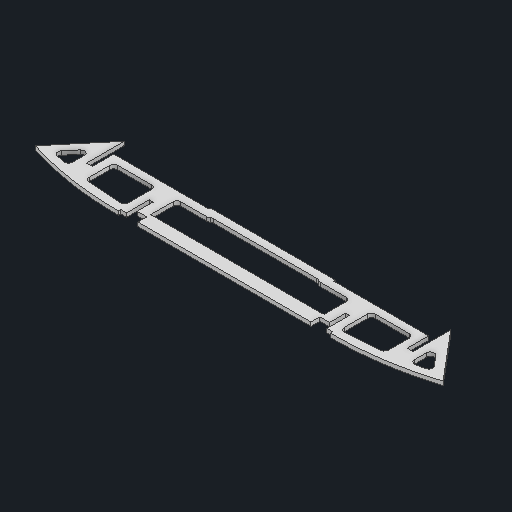
# Autodesk Inventor part: tail_2
Saved by Autodesk Inventor 2023 (Build 270158030, 158C)
## iProperties
Created: 2022-03-21
Part Number: tail_2
Material: Generic
Document SubType Name: Modeling
Designer: kardo
Density: 1 g/cm^3
Appearance: Default
Author: kardo
Autodesk Inventor part; units mm, degrees
ref_plane "YZ Plane" through (0, 0, 0) normal (1, 0, 0) x (0, 1, 0)
ref_plane "XZ Plane" through (0, 0, 0) normal (0, 1, 0) x (-1, 0, 0)
ref_plane "XY Plane" through (0, 0, 0) normal (0, 0, 1) x (1, 0, 0)
derived "parameters_frame.ipt"
derived "stencil_frame.ipt"
sketch "sk_joint_locations" plane through (81.12, 0, 0) normal (1, 0, 0) x (0, 1, 0)
  line L0 (0, 0) -> (111.39, 7.7891) construction
  line L1 (30.81, 28.832) -> (94.8, 28.832) construction
  arc A0 (30.81, 28.832) -> (9.48, 28.5282) centre (30.81, -720.1791) ccw construction
  line L2 (-254.1001, 21.0191) -> (9.48, 28.5282) construction
  line L3 (-363, 18.496) -> (-275.8801, 20.463) construction
  arc A1 (-275.8801, 20.463) -> (-254.1001, 21.0191) centre (-359.1231, 3707.4463) ccw construction
  line L4 (-210.8824, 4616.4994) -> (225.0382, -1617.4555) construction
  line L5 (-242.0001, 4592.9714) -> (-242.0001, -1605.7041) construction
  line L6 (-120.9999, 4592.9714) -> (-120.9999, -1605.7041) construction
  line L7 (-363, 4592.9714) -> (-363, -1605.7041) construction
  line L8 (0, 4592.9714) -> (0, -1605.7041) construction
  line L9 (551.8244, 47.4419) -> (-603.6686, 7.0912) construction
  line L10 (-657.8036, -26.1228) -> (709.4042, 69.4817) construction
  line L11 (178.2183, 30.3929) -> (177.9391, 38.388) construction
  line L12 (185.9231, 36.8959) -> (186.4825, 28.8959) construction
  line L13 (0, 6.528) -> (111.1168, 11.6964) construction
  line L14 (-242.0001, 45.8501) -> (-242.0001, 21.3638) construction
  line L15 (-363, 37.4293) -> (-363, 18.496) construction
  line L16 (-120.9999, 51.0063) -> (-120.9999, 24.811) construction
  line L17 (0, 52.89) -> (0, 28.2581) construction
  line L18 (108.3896, 50.6971) -> (108.935, 42.897) construction
  line L19 (109.4805, 35.0968) -> (108.935, 42.897) construction
  line L20 (109.4805, 35.0968) -> (110.0259, 27.2967) construction
  line L21 (110.0259, 27.2967) -> (110.5713, 19.4965) construction
  line L22 (110.5713, 19.4965) -> (111.1168, 11.6964) construction
  line L23 (0, 6.528) -> (0, 0) construction
  spline S0 degree 4 poles (-363, 37.4293) (-272.3626, 45.1427) (-181.5879, 49.7528) (-90.8131, 52.89) (0, 52.89) knots 0 0 0 0 0 1 1 1 1 1
  spline S1 degree 3 poles (0, 52.89) (86.3106, 52.89) (181.3207, 49.5034) (237, 36.448) knots 0 0 0 0 1 1 1 1
  spline S2 degree 2 poles (111.39, 7.7891) (176.0348, 12.3096) (237, 36.448) knots 0 0 0 1 1 1
  line L24 (94.8, 37.536) -> (94.8, 28.832) construction
  line L25 (94.8, 35.548) -> (94.8, 30.82) construction
  point P0 (-210.8824, 4616.4994)
  point P1 (225.0382, -1617.4555)
  point P2 (178.0787, 34.3904)
  point P3 (186.2028, 32.8959)
  point P4 (134.9575, 11.3411)
  point P5 (-363, 27.9627)
  point P6 (-242.0001, 33.6069)
  point P7 (-120.9999, 37.9086)
  point P8 (0, 40.5741)
  point P9 (94.8, 33.184)
sketch "sk_cowl_joint_locations" plane through (54.6, 0, 0) normal (1, 0, 0) x (0, 1, 0)
  line L0 (-363, 18.496) -> (-275.8801, 20.463) construction
  arc A0 (-275.8801, 20.463) -> (-254.1001, 21.0191) centre (-359.1231, 3707.4463) ccw construction
  line L1 (-254.1001, 21.0191) -> (9.48, 28.5282) construction
  arc A1 (30.81, 28.832) -> (9.48, 28.5282) centre (30.81, -720.1791) ccw construction
  line L2 (30.81, 28.832) -> (94.8, 28.832) construction
  line L3 (94.8, 30.032) -> (30.81, 30.032) construction
  arc A2 (30.81, 30.032) -> (9.4458, 29.7277) centre (30.81, -720.1791) ccw construction
  line L4 (9.4458, 29.7277) -> (-254.1343, 22.2186) construction
  arc A3 (-275.9072, 21.6626) -> (-254.1343, 22.2186) centre (-359.1231, 3707.4463) ccw construction
  line L5 (-275.9072, 21.6626) -> (-363, 19.6963) construction
  line L6 (-242.0001, 4592.9714) -> (-242.0001, -1605.7041) construction
  line L7 (-120.9999, 4592.9714) -> (-120.9999, -1605.7041) construction
  line L8 (-363, 4592.9714) -> (-363, -1605.7041) construction
  line L9 (0, 4592.9714) -> (0, -1605.7041) construction
  line L10 (-242.0001, 45.0688) -> (-242.0001, 22.5643) construction
  line L11 (-120.9999, 49.9661) -> (-120.9999, 26.0115) construction
  line L12 (-363, 19.6963) -> (-363, 19.6963)
  line L13 (-363, 19.6963) -> (-363, 36.9211) construction
  line L14 (-1229.7832, 4422.8213) -> (280.3081, -1633.8241) construction
  line L15 (-362.7741, 36.9211) -> (-363, 39.712) construction
  line L16 (0, 51.6) -> (0, 29.4586) construction
  spline S0 degree 2 poles (-363, 39.712) (-181.6483, 54.394) (0, 54.4) knots 0 0 0 1 1 1
  spline S1 degree 3 poles (0, 54.4) (31.284, 54.4) (68.256, 47.9917) (94.8, 37.536) knots 1 1 1 1 2 2 2 2
  spline S2 degree 3 poles (93.7738, 34.9308) (89.4268, 36.6431) (81.2968, 39.4556) (71.234, 42.2519) (63.4432, 44.1558) (58.1419, 45.3261) (51.4169, 46.6598) (45.9725, 47.6212) (39.1225, 48.6857) (33.6211, 49.4253) (26.7536, 50.2046) (21.2812, 50.7098) (14.5037, 51.1886) (7.8073, 51.5121) (2.5751, 51.6) (0, 51.6) knots 1 1 1 1 1.166667 1.291667 1.333333 1.416667 1.458333 1.541667 1.583333 1.666667 1.708333 1.791667 1.833333 1.916667 2 2 2 2
  spline S3 degree 3 poles (0, 51.6) (-20.1706, 51.5993) (-55.4643, 51.3605) (-95.7903, 50.6123) (-126.0307, 49.8474) (-146.1889, 49.2356) (-171.3841, 48.3435) (-191.5382, 47.528) (-216.7283, 46.3813) (-236.8783, 45.3621) (-262.0632, 43.9608) (-282.2091, 42.7379) (-307.3889, 41.082) (-332.5661, 39.2987) (-352.7052, 37.7363) (-362.7741, 36.9211) knots 0 0 0 0 0.166667 0.291667 0.333333 0.416667 0.458333 0.541667 0.583333 0.666666 0.708333 0.791666 0.833333 0.916666 1 1 1 1
  line L17 (-142.5135, 45.4866) -> (-137.5404, 25.5402) construction
  line L18 (-134.9025, 31.4945) -> (-138.7836, 30.5268) construction
  line L19 (-137.3891, 41.4677) -> (-141.2702, 40.5) construction
  line L20 (-142.5135, 45.4866) -> (-138.6324, 46.4543) construction
  line L21 (-137.5404, 25.5402) -> (-133.6592, 26.5079) construction
  line L22 (-138.6324, 46.4543) -> (-138.8117, 52.2515) construction
  point P0 (0, 0)
  point P1 (-363, 28.3087)
  point P2 (-242.0001, 33.8165)
  point P3 (-120.9999, 37.9888)
  point P4 (0, 40.5293)
  point P5 (-1229.7832, 4422.8213)
  point P6 (280.3081, -1633.8241)
  point P7 (-85.2629, 50.788)
  point P8 (0, 40.5293)
sketch "sk_tail_2_base" plane through (0, -242.0001, 0) normal (0, 1, 0) x (-1, 0, 0)
  spline S0 degree 2 poles (-54.6, 47.8729) (-109.262, 47.8729) (-156, 14.7183) knots 0 0 0 1 1 1 construction
  line L0 (0, 47.8729) -> (-54.6, 47.8729) construction
  line L1 (760.5328, -994.3388) -> (-2384.0852, 2753.2711) construction
  line L2 (0, -1605.7041) -> (0, 4592.9714) construction
  line L3 (0, 21.7168) -> (-32.32, 21.7168)
  line L4 (-32.32, 21.7168) -> (-32.32, 22.5638)
  line L5 (-32.32, 22.5638) -> (-81.12, 22.5638)
  line L6 (-81.12, 22.5638) -> (-81.12, 33.6069)
  line L7 (-81.12, 33.6069) -> (-84.12, 33.6069)
  line L8 (-84.12, 33.6069) -> (-84.12, 14.1461)
  line L9 (-84.12, 14.1461) -> (-105.0165, 39.0496)
  line L10 (0, 46.6729) -> (-54.6, 46.6729)
  line L11 (0, 46.6729) -> (0, 21.7168)
  spline S1 degree 5 poles (-54.6, 46.6729) (-65.235, 46.6727) (-75.8695, 45.884) (-86.4273, 44.246) (-107.4395, 39.1871) (-127.368, 30.8129) (-137.094, 25.7751) (-146.4079, 20.0514) (-155.3057, 13.7395) knots 0 0 0 0 0 0 0.493638 0.493638 0.493638 1 1 1 1 1 1
  point P0 (0, 0)
  point P1 (-34.32, 21.3638)
  point P2 (-34.32, 20.5168)
  dimension "d3" = 1.2
  dimension "d4" = 1.2
  dimension "d5" = 1.2
  dimension "d6" = 2
  dimension "d7" = 3
  dimension "d8" = 1.2
  constraints: 18 end point, 5 parallel, 4 perpendicular, 2 point on line, 1 coincident, 4 other
  measures "d4" distance from line of L3 point (-34.32, 20.517)
  measures "d5" distance from line of L5 point (-34.32, 21.364)
  measures "d6" distance from line of point (-34.32, 21.364) L4
  measures "d7" distance of L6.end L7.end
  measures "d8" distance between parallel lines of L1 L9
extrude "thicken" add sketch "sk_tail_2_base" along normal blind 2
sketch "sk_cut_joint" plane through (0, -242.0001, 0) normal (0, 1, 0) x (-1, 0, 0)
  line L0 (0, 47.8729) -> (-54.6, 47.8729) projected
  line L1 (-54.6, -1605.7041) -> (-54.6, 4592.9714) construction
  line L2 (-49.6, 47.8729) -> (-49.6, 33.8165)
  line L3 (-49.6, 33.8165) -> (-51.6, 33.8165)
  line L4 (-51.6, 33.8165) -> (-51.6, 47.8729)
  point P0 (0, 0)
  point P1 (-54.6, 33.8165)
  dimension "d11" = 5
  dimension "d12" = 2
  constraints: 6 end point, 3 parallel, 3 point on line
  measures "d11" distance between parallel lines of L1 L2
  measures "d12" distance between parallel lines of L2 L4
extrude "cut_joint" cut sketch "sk_cut_joint" along normal through all both and the other way through all
sketch "sk_cut_liner" plane through (0, -242.0001, 0) normal (0, 1, 0) x (-1, 0, 0)
  line L0 (0, 47.8729) -> (-54.6, 47.8729) projected
  line L1 (-54.6, -1605.7041) -> (-54.6, 4592.9714) projected
  line L2 (-44.6, 47.8729) -> (-44.6, 42.0729)
  line L3 (-44.6, 42.0729) -> (-49.6, 42.0729)
  line L4 (-49.6, 42.0729) -> (-49.6, 45.4729)
  line L5 (-49.6, 45.4729) -> (-54.6, 45.4729)
  point P0 (0, 0)
  dimension "d14" = 2.4
  dimension "d15" = 5
  dimension "d17" = 5
  dimension "d40" = 5.8
  constraints: 8 end point, 4 parallel, 2 point on line
  measures "d14" distance between parallel lines of L0 L5
  measures "d15" distance between parallel lines of L1 L4
  measures "d17" distance between parallel lines of L2 L4
  measures "d40" distance of L2.start L2.end
extrude "cut_liner" cut sketch "sk_cut_liner" along normal through all both and the other way through all
sketch "sk_cut_weight" plane through (0, -242.0001, 0) normal (0, 1, 0) x (-1, 0, 0)
  line L0 (-44.6, 47.8729) -> (-44.6, 42.0729) construction
  line L1 (-44.6, 42.0729) -> (-49.6, 42.0729) construction
  line L2 (-49.6, 42.0729) -> (-49.6, 45.4729) projected
  line L3 (-32.32, 22.5638) -> (-81.12, 22.5638) construction
  line L4 (-32.32, 21.7168) -> (-32.32, 22.5638) construction
  line L5 (0, 21.7168) -> (-32.32, 21.7168) construction
  line L6 (-81.12, 22.5638) -> (-81.12, 33.6069) construction
  line L7 (-84.12, 33.6069) -> (-84.12, 14.1461) construction
  spline S0 degree 3 poles (-54.6, 46.6729) (-57.6166, 46.6729) (-63.6125, 46.5204) (-71.0149, 45.9488) (-78.3481, 45.0915) (-84.1595, 44.1772) (-91.3552, 42.7486) (-97.057, 41.3771) (-104.1161, 39.3771) (-109.709, 37.5484) (-116.6326, 34.9765) (-122.1174, 32.6902) (-130.2638, 28.9171) (-140.9825, 23.2754) (-150.1426, 17.4021) (-155.3057, 13.7395) knots 0 0 0 0 0.083333 0.166667 0.208333 0.291667 0.333333 0.416667 0.458333 0.541667 0.583333 0.666667 0.708333 0.833333 1 1 1 1 construction
  line L8 (-84.12, 14.1461) -> (-105.0165, 39.0496) construction
  line L9 (0, -1605.7041) -> (0, 4592.9714) projected
  line L10 (-88.12, 25.136) -> (-88.12, 39.3855)
  line L11 (-88.12, 39.3855) -> (-98.2721, 37.2349)
  line L12 (-98.2721, 37.2349) -> (-88.12, 25.136)
  line L13 (-88.12, 39.3855) -> (-88.12, 43.3855) construction
  line L14 (-98.2721, 37.2349) -> (-100.8433, 40.299) construction
  line L15 (0, 40.0729) -> (-44.6, 40.0729)
  line L16 (-44.6, 40.0729) -> (-44.6, 26.5638)
  line L17 (-44.6, 26.5638) -> (-28.32, 26.5638)
  line L18 (-28.32, 26.5638) -> (-28.32, 25.7168)
  line L19 (-28.32, 25.7168) -> (0, 25.7168)
  line L20 (-55.6, 42.6729) -> (-77.12, 41.185)
  line L21 (-77.12, 41.185) -> (-77.12, 26.5638)
  line L22 (-77.12, 26.5638) -> (-55.6, 26.5638)
  line L23 (-55.6, 26.5638) -> (-55.6, 42.6729)
  line L24 (-49.6, 42.0729) -> (-49.6, 22.5638) construction
  line L25 (-49.6, 42.0729) -> (-51.6, 42.0729) construction
  line L26 (-51.6, 42.0729) -> (-51.6, 22.5638) construction
  line L27 (-77.12, 41.185) -> (-77.3959, 45.1755) construction
  point P0 (0, 0)
  dimension "d22" = 2
  dimension "d23" = 4
  dimension "d24" = 4
  dimension "d25" = 4
  dimension "d26" = 4
  dimension "d28" = 4
  dimension "d29" = 4
  dimension "d30" = 4
  dimension "d31" = 4
  dimension "d32" = 4
  dimension "d33" = 4
  dimension "d34" = 4
  dimension "d35" = 2
  dimension "d39" = 4
  constraints: 36 end point, 11 parallel, 4 collinear, 4 point on line, 2 perpendicular, 3 other
  measures "d22" distance between parallel lines of L24 L26
  measures "d23" distance between parallel lines of L23 L26
  measures "d24" distance between parallel lines of L3 L22
  measures "d25" distance between parallel lines of L6 L21
  measures "d26" distance of L20.end L27.end
  measures "d28" distance between parallel lines of L7 L10
  measures "d29" distance between parallel lines of L8 L12
  measures "d30" distance of L10.end L13.end
  measures "d31" distance of L11.end L14.end
  measures "d32" distance between parallel lines of L5 L19
  measures "d33" distance between parallel lines of L4 L18
  measures "d34" distance between parallel lines of L3 L17
  measures "d35" distance between parallel lines of L1 L15
  measures "d39" vertical distance of L20.start point (-54.6, 46.673)
extrude "cut_weight" cut sketch "sk_cut_weight" along normal through all both and the other way through all
fillet "rounding" radius 2 10 edges at (28.32, -241.0001, 26.5638) (28.32, -241.0001, 25.7168) (44.6, -241.0001, 26.5638) (77.12, -241.0001, 41.185) (98.2721, -241.0001, 37.2349) (77.12, -241.0001, 26.5638) (88.12, -241.0001, 25.136) (55.6, -241.0001, 26.5638) (55.6, -241.0001, 42.6729) (88.12, -241.0001, 39.3855)
mirror "mirror" about plane through (0, 0, 0) normal (1, 0, 0)
equation "\"d3\" = shell_thickness"
equation "\"d4\" = shell_thickness"
equation "\"d5\" = shell_thickness"
equation "\"d6\" = bulkhead_thickness"
equation "\"d7\" = stringer_thickness"
equation "\"d8\" = shell_thickness"
equation "\"d9\" = bulkhead_thickness"
equation "\"d11\" = cowl_liner_width"
equation "\"d12\" = bulkhead_thickness"
equation "\"d14\" = shell_thickness + cowl_liner_thickness"
equation "\"d15\" = cowl_liner_width"
equation "\"d17\" = cowl_sealing_width"
equation "\"d40\" = cowl_sealing_thickness + cowl_shell_thickness + cowl_liner_thickness"
equation "\"d22\" = bulkhead_thickness"
equation "\"d23\" = bulkhead_inset"
equation "\"d24\" = bulkhead_inset"
equation "\"d25\" = bulkhead_inset"
equation "\"d26\" = bulkhead_inset"
equation "\"d28\" = bulkhead_inset"
equation "\"d29\" = bulkhead_inset"
equation "\"d30\" = bulkhead_inset"
equation "\"d31\" = bulkhead_inset"
equation "\"d32\" = bulkhead_inset"
equation "\"d33\" = bulkhead_inset"
equation "\"d34\" = bulkhead_inset"
equation "\"d39\" = bulkhead_inset"
equation "\"d38\" = 0.5 * bulkhead_inset"
equation "\"shell_thickness\" = 1.2"
equation "\"stringer_thickness\" = 3"
equation "\"bulkhead_thickness\" = 2"
equation "\"cowl_liner_width\" = 5"
equation "\"cowl_liner_thickness\" = 1.2"
equation "\"cowl_sealing_width\" = 5"
equation "\"cowl_sealing_thickness\" = 3"
equation "\"cowl_shell_thickness\" = 1.6"
equation "\"bulkhead_inset\" = 4"
body "Solid1"
